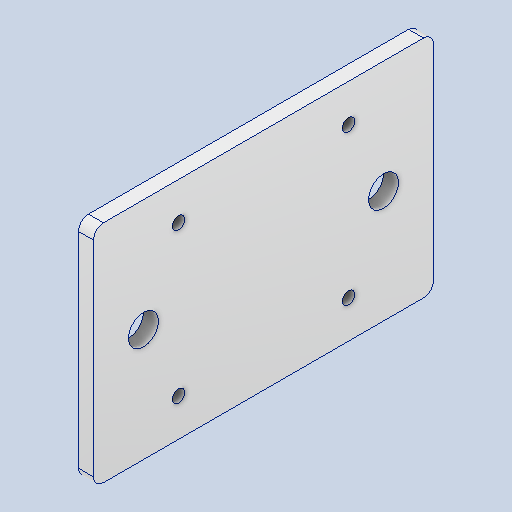
# Autodesk Inventor part: belt_liner_v2_Plate_12
Saved by Autodesk Inventor 2025.2 (Build 292293000, 293)
## iProperties
Created: 2025-01-06
Part Number: belt_liner_v2_Plate_12
Material: アルミニウム 6061
Document SubType Name: Modeling
Designer: haruy
Density: 2.7 g/cm^3
Appearance: アルミニウム - フラット
Author: haruy
Autodesk Inventor part; units mm, degrees
ref_plane "YZ Plane" through (0, 0, 0) normal (1, 0, 0) x (0, 1, 0)
ref_plane "XZ Plane" through (0, 0, 0) normal (0, 1, 0) x (-1, 0, 0)
ref_plane "XY Plane" through (0, 0, 0) normal (0, 0, 1) x (1, 0, 0)
sketch "スケッチ1" plane through (0, 0, 0) normal (1, 0, 0) x (0, 1, 0)
  line L0 (131.4398, 116.9683) -> (131.4398, -135.5317)
  line L1 (131.4398, 116.9683) -> (116.4398, 116.9683)
  circle A0 centre (138.9398, 63.9683) radius 3
  circle A1 centre (138.9398, 15.9683) radius 3
  line L2 (116.4398, 73.9683) -> (161.4398, 73.9683)
  line L3 (161.4398, -135.5317) -> (161.4398, 116.9683)
  line L4 (116.4398, 5.9683) -> (161.4398, 5.9683)
  line L5 (116.4398, 116.9683) -> (116.4398, -135.5317)
  line L6 (116.4398, 39.9683) -> (161.4398, 39.9683)
  circle A2 centre (123.9398, 22.9683) radius 1.25
  circle A3 centre (123.9398, 56.9683) radius 1.25
  line L7 (138.9398, 63.9683) -> (138.9398, 15.9683)
  circle A4 centre (153.9398, 56.9683) radius 1.25
  circle A5 centre (153.9398, 22.9683) radius 1.25
  line L8 (116.4398, 73.9683) -> (116.4398, 5.9683)
  line L9 (161.4398, 5.9683) -> (161.4398, 73.9683)
  point P0 (0, 0)
  point P1 (-153.5602, 148.7156)
  point P2 (138.9398, 39.9683)
  point P3 (123.9398, 116.9683)
  dimension "d0" = 7.5
  dimension "d1" = 77
  dimension "d2" = 6
  dimension "d3" = 6
  dimension "d4" = 48
  dimension "d5" = 24
  dimension "d6" = 7.5
  dimension "d7" = 7.5
  dimension "d8" = 10
  dimension "d9" = 10
  dimension "d10" = 34
  dimension "d11" = 2.5
  dimension "d12" = 2.5
  dimension "d13" = 17
  dimension "d14" = 17
  dimension "d15" = 7.5
  dimension "d16" = 7.5
  constraints: 20 end point, 6 centre point, 4 point on line, 2 horizontal, 2 symmetric about line, 1 collinear, 1 midpoint, 1 parallel, 1 vertical, 2 other
  measures "d0" distance from line of L0 point (138.94, 39.968)
  measures "d1" vertical distance of point (123.94, 116.968) point (138.94, 39.968)
  measures "d2" diameter of A0
  measures "d3" diameter of A1
  measures "d4" distance of L7.end L7.start
  measures "d5" distance of point (138.94, 39.968) L7.start
  measures "d6" distance from line of L7.start L0
  measures "d7" distance from line of L0 L7.end
  measures "d8" distance from line of L7.end L4
  measures "d9" distance from line of L7.start L2
  measures "d10" distance between parallel lines of L4 L6
  measures "d11" diameter of A2
  measures "d12" diameter of A3
  measures "d13" distance from line of L6 A2.centre
  measures "d14" distance from line of A3.centre L6
  measures "d15" distance from line of A3.centre L5
  measures "d16" distance from line of L5 A2.centre
extrude "押し出し1" add sketch "スケッチ1" against normal blind 3 contours L2 L3 L6 L0 | L0 L6 L5 L2 | L6 L3 L4 L0 | L0 L4 L5 L6
fillet "フィレット1" radius 2 4 edges at (-1.5, 161.4398, 73.9683) (-1.5, 116.4398, 73.9683) (-1.5, 116.4398, 5.9683) (-1.5, 161.4398, 5.9683)
equation "\"d6\" = d0"
equation "\"d7\" = d0"
equation "\"d14\" = d13"
equation "\"d15\" = d0"
equation "\"d16\" = d0"
